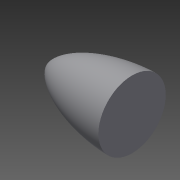
# Autodesk Inventor part: moncong
Saved by Autodesk Inventor 2014 SP1 (Build 180222100, 222)
## iProperties
Created: 2018-05-14
Part Number: moncong
Material: Generic
Document SubType Name: Modeling
Designer: Dadang
Density: 1 g/cm^3
Appearance: Default
Author: Dadang
Autodesk Inventor part; units mm, degrees
ref_plane "YZ Plane" through (0, 0, 0) normal (1, 0, 0) x (0, 1, 0)
ref_plane "XZ Plane" through (0, 0, 0) normal (0, 1, 0) x (-1, 0, 0)
ref_plane "XY Plane" through (0, 0, 0) normal (0, 0, 1) x (1, 0, 0)
sketch "Sketch1" plane through (0, 0, 0) normal (0, 0, 1) x (1, 0, 0)
  line L0 (0, 0) -> (100, 0)
  line L1 (100, 0) -> (100, 40)
  line L2 (0, 0) -> (1.6697, 12.0016) construction
  line L3 (1.6697, 12.0016) -> (28.6574, 34.7725) construction
  line L4 (28.6574, 34.7725) -> (80.7775, 40) construction
  line L5 (80.7775, 40) -> (100, 40) construction
  spline S0 degree 4 poles (0, 0) (1.6697, 12.0016) (28.6574, 34.7725) (80.7775, 40) (100, 40) knots 1 1 1 1 1 2 2 2 2 2
  dimension "d0" = 100
  dimension "d1" = 40
  constraints: 4 end point, 1 horizontal, 1 parallel, 1 perpendicular, 3 other
  measures "d0" distance of L0.start L0.end
  measures "d1" distance of L0.end L1.end
revolve "Revolution1" add sketch "Sketch1" angle 360 about axis through (0, 0, 0) along (1, 0, 0)
body "Solid1"
